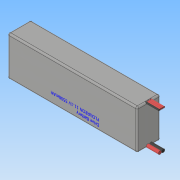
# Autodesk Inventor part: DriveBattery
Saved by Autodesk Inventor 2017.3 (Build 213256000, 256)
## iProperties
Created: 2018-01-30
Part Number: DriveBattery
Material: ABS Plastic
Document SubType Name: Modeling
Designer: Derek Wider
Density: 1.77812 g/cm^3
Appearance: Light Gray
Mass: 396.893 g
Surface Area: 275.416 cm^2
Volume: 223.209 cm^3
Author: Derek Wider
Autodesk Inventor part; units mm, degrees
ref_plane "YZ Plane" through (0, 0, 0) normal (1, 0, 0) x (0, 1, 0)
ref_plane "XZ Plane" through (0, 0, 0) normal (0, 1, 0) x (-1, 0, 0)
ref_plane "XY Plane" through (0, 0, 0) normal (0, 0, 1) x (1, 0, 0)
sketch "Sketch1" plane through (0, 0, 0) normal (0, 0, 1) x (1, 0, 0)
  line L0 (0, 0) -> (160, 0)
  line L1 (160, 0) -> (160, 49)
  line L2 (160, 49) -> (0, 49)
  line L3 (0, 49) -> (0, 0)
  dimension "d0" = 160
  dimension "d1" = 49
  constraints: 8 end point, 2 parallel, 1 horizontal, 1 perpendicular
  measures "d0" distance of L1.end L2.end
  measures "d1" distance of L0.end L1.end
extrude "Extrusion1" add sketch "Sketch1" along normal blind 28.5
fillet "Fillet1" radius 2 12 edges at (80, 49, 28.5) (0, 49, 14.25) (80, 49, 0) (0, 24.5, 28.5) (80, 0, 28.5) (0, 0, 14.25) (0, 24.5, 0) (160, 24.5, 28.5) (160, 0, 14.25) (160, 24.5, 0) (160, 49, 14.25) (80, 0, 0)
sketch "Sketch2" plane through (0, 0, 28.5) normal (0, 0, 1) x (1, 0, 0)
  line L0 (112.9507, 4.761) -> (47.847, 4.761) construction
  line L1 (47.847, 4.761) -> (47.847, 21.3737) construction
  line L2 (47.847, 21.3737) -> (112.9507, 21.3737) construction
  line L3 (112.9507, 21.3737) -> (112.9507, 4.761) construction
  constraints: 2 other
sketch "Sketch3" plane through (160, 2, 2) normal (1, 0, 0) x (0, 0, -1)
  line L0 (-24.5, -2) -> (0, -2) projected
  line L1 (0, 47) -> (-24.5, 47) projected
  circle A0 centre (-13.5, 0) radius 2
  circle A1 centre (-9.5, 0) radius 2
  circle A2 centre (-14.5, 46) radius 1
  circle A3 centre (-12.5, 46) radius 1
  circle A4 centre (-10.5, 46) radius 1
  circle A5 centre (-8.5, 46) radius 1
  line L2 (-26.5, 45) -> (-26.5, 0) projected
  point P0 (2, -2)
  dimension "d5" = 4
  dimension "d6" = 4
  dimension "d7" = 2
  dimension "d8" = 2
  dimension "d9" = 2
  dimension "d10" = 2
  dimension "d11" = 12
  dimension "d12" = 13
  constraints: 10 tangent, 6 centre point
  measures "d5" diameter of A0
  measures "d6" diameter of A1
  measures "d7" diameter of A2
  measures "d8" diameter of A3
  measures "d9" diameter of A4
  measures "d10" diameter of A5
  measures "d11" distance from line of A2.centre L2
  measures "d12" distance from line of L2 A0.centre
extrude "Extrusion2" add sketch "Sketch3" along normal blind 15 and the other way blind 3 contours A0 | A1 | A5 | A4 | A3 | A2
body "Solid1"
